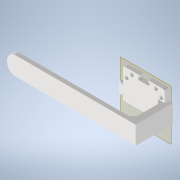
# Autodesk Inventor part: 40_Cube_XY_Table_Illumination_Arm
Saved by Autodesk Inventor 2022 (Build 260153000, 153)
## iProperties
Created: 2022-09-09
Part Number: 40_Cube_XY_Table_Illumination_Arm
Material: Generisch
Document SubType Name: Modeling
Designer: UC2
Density: 1 g/cm^3
Appearance: Vorgabe
Author: UC2
Autodesk Inventor part; units mm, degrees
ref_plane "YZ Plane" through (0, 0, 0) normal (1, 0, 0) x (0, 1, 0)
ref_plane "XZ Plane" through (0, 0, 0) normal (0, 1, 0) x (-1, 0, 0)
ref_plane "XY Plane" through (0, 0, 0) normal (0, 0, 1) x (1, 0, 0)
ref_plane "Arbeitsebene1" through (0, 0, 0) normal (0, 0, 1) x (1, 0, 0)
sketch "Skizze1" plane through (0, 0, 0) normal (0, 0, 1) x (1, 0, 0)
  circle A0 centre (-6.0705, 15.2895) radius 3.5 projected
  circle A1 centre (15.2895, -6.0705) radius 3.5 projected
  line L0 (30.5395, 32.5395) -> (0.0395, 32.5395) projected
  arc A2 (32.5395, 30.5395) -> (30.5395, 32.5395) centre (30.5395, 30.5395) ccw projected
  line L1 (32.5395, 30.5395) -> (32.5395, 0.0395) projected
  arc A3 (30.5395, -1.9605) -> (32.5395, 0.0395) centre (30.5395, 0.0395) ccw projected
  line L2 (0.0395, -1.9605) -> (30.5395, -1.9605) projected
  arc A4 (-1.9605, 0.0395) -> (0.0395, -1.9605) centre (0.0395, 0.0395) ccw projected
  line L3 (-1.9605, 0.0395) -> (-1.9605, 30.5395) projected
  arc A5 (0.0395, 32.5395) -> (-1.9605, 30.5395) centre (0.0395, 30.5395) ccw projected
  circle A6 centre (-4.7105, -4.7105) radius 2.45 projected
  circle A7 centre (0.7895, -5.5105) radius 2.3 projected
  circle A8 centre (-5.5105, 0.7895) radius 2.3 projected
  circle A9 centre (-5.5105, 29.7895) radius 2.3 projected
  circle A10 centre (0.7895, 36.0895) radius 2.3 projected
  circle A11 centre (-4.7105, 35.2895) radius 2.45 projected
  circle A12 centre (36.0895, 0.7895) radius 2.3 projected
  circle A13 centre (29.7895, -5.5105) radius 2.3 projected
  circle A14 centre (35.2895, -4.7105) radius 2.45 projected
  circle A15 centre (36.0895, 29.7895) radius 2.3 projected
  circle A16 centre (29.7895, 36.0895) radius 2.3 projected
  circle A17 centre (35.2895, 35.2895) radius 2.45 projected
  line L4 (20.4019, 40.2895) -> (20.4019, 39.1582) projected
  arc A18 (20.4019, 39.1582) -> (20.6778, 38.7524) centre (20.7437, 39.0939) ccw projected
  arc A19 (20.2895, 34.6895) -> (20.6778, 38.7524) centre (20.2895, 36.7395) ccw projected
  line L5 (20.2895, 34.6895) -> (10.1895, 34.6895) projected
  arc A20 (9.8548, 38.762) -> (10.1895, 34.6895) centre (10.1895, 36.7395) ccw projected
  arc A21 (9.8548, 38.762) -> (10.1895, 39.1567) centre (9.7895, 39.1567) ccw projected
  line L6 (10.1895, 39.1567) -> (10.1895, 40.2895) projected
  line L7 (10.1895, 40.2895) -> (-7.7105, 40.2895) projected
  arc A22 (-7.7105, 40.2895) -> (-9.7105, 38.2895) centre (-7.7105, 38.2895) ccw projected
  line L8 (-9.7105, 20.2895) -> (-9.7105, 38.2895) projected
  line L9 (-10.8433, 20.2895) -> (-9.7105, 20.2895) projected
  arc A23 (-11.3366, 20.7079) -> (-10.8433, 20.2895) centre (-10.8433, 20.7895) ccw projected
  arc A24 (-11.3366, 20.7079) -> (-15.2105, 20.3895) centre (-13.2605, 20.3895) ccw projected
  line L10 (-15.2105, 10.2895) -> (-15.2105, 20.3895) projected
  arc A25 (-15.2105, 10.2895) -> (-11.3515, 9.8916) centre (-13.2605, 10.2895) ccw projected
  arc A26 (-10.862, 10.2895) -> (-11.3515, 9.8916) centre (-10.862, 9.7895) ccw projected
  line L11 (-9.7105, 10.2895) -> (-10.862, 10.2895) projected
  line L12 (-9.7105, -7.7105) -> (-9.7105, 10.2895) projected
  arc A27 (-9.7105, -7.7105) -> (-7.7105, -9.7105) centre (-7.7105, -7.7105) ccw projected
  line L13 (-7.7105, -9.7105) -> (10.2895, -9.7105) projected
  line L14 (10.2895, -10.8433) -> (10.2895, -9.7105) projected
  arc A28 (9.8712, -11.3366) -> (10.2895, -10.8433) centre (9.7895, -10.8433) ccw projected
  arc A29 (9.8712, -11.3366) -> (10.1895, -15.2105) centre (10.1895, -13.2605) ccw projected
  line L15 (20.2895, -15.2105) -> (10.1895, -15.2105) projected
  arc A30 (20.2895, -15.2105) -> (20.6875, -11.3515) centre (20.2895, -13.2605) ccw projected
  arc A31 (20.2895, -10.862) -> (20.6875, -11.3515) centre (20.7895, -10.862) ccw projected
  line L16 (20.2895, -9.7105) -> (20.2895, -10.862) projected
  line L17 (20.2895, -9.7105) -> (38.2895, -9.7105) projected
  arc A32 (38.2895, -9.7105) -> (40.2895, -7.7105) centre (38.2895, -7.7105) ccw projected
  line L18 (40.2895, 10.1772) -> (40.2895, -7.7105) projected
  line L19 (40.2895, 10.1772) -> (39.1582, 10.1772) projected
  arc A33 (39.1582, 10.1772) -> (38.7524, 9.9013) centre (39.0939, 9.8354) ccw projected
  arc A34 (34.6895, 10.2895) -> (38.7524, 9.9013) centre (36.7395, 10.2895) ccw projected
  line L20 (34.6895, 10.2895) -> (34.6895, 20.3895) projected
  arc A35 (38.762, 20.7242) -> (34.6895, 20.3895) centre (36.7395, 20.3895) ccw projected
  arc A36 (38.762, 20.7242) -> (39.1567, 20.3895) centre (39.1567, 20.7895) ccw projected
  line L21 (39.1567, 20.3895) -> (40.2895, 20.3895) projected
  line L22 (40.2895, 38.2895) -> (40.2895, 20.3895) projected
  arc A37 (40.2895, 38.2895) -> (38.2895, 40.2895) centre (38.2895, 38.2895) ccw projected
  line L23 (38.2895, 40.2895) -> (20.4019, 40.2895) projected
  line L24 (40.2895, 26.3895) -> (45.2895, 26.3895)
  line L25 (45.2895, 26.3895) -> (45.2895, 4.1772)
  line L26 (45.2895, 4.1772) -> (40.2895, 4.1772)
  line L27 (40.2895, 4.1772) -> (40.2895, 26.3895)
  point P0 (0, 0)
  dimension "d0" = 5
  dimension "d2" = 6
  dimension "d3" = 6
  constraints: 8 end point, 2 parallel, 1 horizontal, 1 perpendicular, 1 point on line
  measures "d0" distance of L25.end L26.end
  measures "d2" distance of L21.end L24.start
  measures "d3" distance between parallel lines of L26 L19
extrude "Extrusion1" add sketch "Skizze1" along normal blind 5 contours A0 | A2 L1 A3 L2 A4 L3 A5 L0 | A6 | A11 | A14 | A17 | L23 A37 L22 L21 A36 A35 L20 A34 A33 L19 L18 A32 L17 L16 A31 A30 L15 A29 A28 L14 L13 A27 L12 L11 A26 A25 L10 A24 A23 L9 L8 A22 L7 L6 A21 A20 L5 A19 A18 L4 | L24 L25 L26 L18 L27 L22 | L27 L19 A33 A34 L20 A35 A36 L21
chamfer "Fase1" distance 1 angle 45 8 edges at (-1.5105, 36.0895, 0) (27.4895, 36.0895, 0) (33.7895, 29.7895, 0) (33.7895, 0.7895, 0) (27.4895, -5.5105, 0) (-1.5105, -5.5105, 0) (-7.8105, 0.7895, 0) (-7.8105, 29.7895, 0)
sketch "Skizze2" plane through (0, 0, 5) normal (0, 0, 1) x (1, 0, 0)
  line L0 (40.2895, 4.1772) -> (45.2895, 4.1772) projected
  line L1 (45.2895, 26.3895) -> (40.2895, 26.3895) projected
  line L2 (45.2895, 4.1772) -> (37.2895, 4.1772)
  line L3 (37.2895, 4.1772) -> (37.2895, 26.3895)
  line L4 (37.2895, 26.3895) -> (45.2895, 26.3895)
  line L5 (45.2895, 26.3895) -> (45.2895, 4.1772)
  point P0 (0, 0)
  point P1 (45.2895, 26.3895)
  point P2 (40.2895, 4.1772)
  dimension "d9" = 8
  constraints: 8 end point, 2 parallel, 1 horizontal, 1 perpendicular, 1 point on line
  measures "d9" distance of L3.end L4.end
extrude "Extrusion2" add sketch "Skizze2" along normal blind 45
sketch "Skizze3" plane through (0, 0, 50) normal (0, 0, 1) x (1, 0, 0)
  line L0 (45.2895, 26.3895) -> (37.2895, 26.3895) projected
  line L1 (37.2895, 26.3895) -> (37.2895, 4.1772) projected
  line L2 (37.2895, 4.1772) -> (45.2895, 4.1772) projected
  line L3 (45.2895, 4.1772) -> (45.2895, 26.3895) projected
  line L4 (45.2895, 26.3895) -> (37.2895, 26.3895) projected
  line L5 (37.2895, 26.3895) -> (-109.7105, 26.3895)
  line L6 (-109.7105, 26.3895) -> (-109.7105, 4.1772)
  line L7 (-109.7105, 4.1772) -> (37.2895, 4.1772)
  line L8 (37.2895, 4.1772) -> (37.2895, 26.3895)
  circle A0 centre (36.0895, 29.7895) radius 2.3 projected
  circle A1 centre (29.7895, -5.5105) radius 2.3 projected
  circle A2 centre (0.7895, 36.0895) radius 2.3 projected
  circle A3 centre (-5.5105, 29.7895) radius 2.3 projected
  circle A4 centre (-5.5105, 0.7895) radius 2.3 projected
  circle A5 centre (0.7895, -5.5105) radius 2.3 projected
  circle A6 centre (15.2895, -6.0705) radius 3.5 projected
  circle A7 centre (36.0895, 0.7895) radius 2.3 projected
  circle A8 centre (29.7895, 36.0895) radius 2.3 projected
  arc A9 (40.2895, 38.2895) -> (38.2895, 40.2895) centre (38.2895, 38.2895) ccw projected
  line L9 (38.2895, 40.2895) -> (20.4019, 40.2895) projected
  line L10 (20.4019, 40.2895) -> (20.4019, 39.1582) projected
  arc A10 (20.4019, 39.1582) -> (20.6778, 38.7524) centre (20.7437, 39.0939) ccw projected
  arc A11 (20.2895, 34.6895) -> (20.6778, 38.7524) centre (20.2895, 36.7395) ccw projected
  line L11 (20.2895, 34.6895) -> (10.1895, 34.6895) projected
  arc A12 (9.8548, 38.762) -> (10.1895, 34.6895) centre (10.1895, 36.7395) ccw projected
  arc A13 (9.8548, 38.762) -> (10.1895, 39.1567) centre (9.7895, 39.1567) ccw projected
  line L12 (10.1895, 39.1567) -> (10.1895, 40.2895) projected
  line L13 (10.1895, 40.2895) -> (-7.7105, 40.2895) projected
  arc A14 (-7.7105, 40.2895) -> (-9.7105, 38.2895) centre (-7.7105, 38.2895) ccw projected
  line L14 (-9.7105, 38.2895) -> (-9.7105, 20.2895) projected
  line L15 (-9.7105, 20.2895) -> (-10.8433, 20.2895) projected
  arc A15 (-11.3366, 20.7079) -> (-10.8433, 20.2895) centre (-10.8433, 20.7895) ccw projected
  arc A16 (-11.3366, 20.7079) -> (-15.2105, 20.3895) centre (-13.2605, 20.3895) ccw projected
  line L16 (-15.2105, 20.3895) -> (-15.2105, 10.2895) projected
  arc A17 (-15.2105, 10.2895) -> (-11.3515, 9.8916) centre (-13.2605, 10.2895) ccw projected
  arc A18 (-10.862, 10.2895) -> (-11.3515, 9.8916) centre (-10.862, 9.7895) ccw projected
  line L17 (-10.862, 10.2895) -> (-9.7105, 10.2895) projected
  line L18 (-9.7105, 10.2895) -> (-9.7105, -7.7105) projected
  arc A19 (-9.7105, -7.7105) -> (-7.7105, -9.7105) centre (-7.7105, -7.7105) ccw projected
  line L19 (-7.7105, -9.7105) -> (10.2895, -9.7105) projected
  line L20 (10.2895, -9.7105) -> (10.2895, -10.8433) projected
  arc A20 (9.8712, -11.3366) -> (10.2895, -10.8433) centre (9.7895, -10.8433) ccw projected
  arc A21 (9.8712, -11.3366) -> (10.1895, -15.2105) centre (10.1895, -13.2605) ccw projected
  line L21 (10.1895, -15.2105) -> (20.2895, -15.2105) projected
  arc A22 (20.2895, -15.2105) -> (20.6875, -11.3515) centre (20.2895, -13.2605) ccw projected
  arc A23 (20.2895, -10.862) -> (20.6875, -11.3515) centre (20.7895, -10.862) ccw projected
  line L22 (20.2895, -10.862) -> (20.2895, -9.7105) projected
  line L23 (20.2895, -9.7105) -> (38.2895, -9.7105) projected
  arc A24 (38.2895, -9.7105) -> (40.2895, -7.7105) centre (38.2895, -7.7105) ccw projected
  line L24 (40.2895, -7.7105) -> (40.2895, 4.1772) projected
  line L25 (37.2895, 4.1772) -> (37.2895, 26.3895) projected
  line L26 (40.2895, 26.3895) -> (40.2895, 38.2895) projected
  line L27 (37.2895, 26.3895) -> (40.2895, 26.3895) projected
  line L28 (40.2895, 4.1772) -> (37.2895, 4.1772) projected
  point P0 (0, 0)
  dimension "d24" = 100
  constraints: 8 end point, 2 parallel, 1 horizontal, 1 perpendicular
  measures "d24" distance between parallel lines of L14 L6
extrude "Extrusion3" add sketch "Skizze3" along normal blind 5 contours L3 L2 L1 L0 | L1 L7 L18 L17 A18 A17 L16 A16 A15 L15 L14 L5 | L14 L15 A15 A16 L16 A17 A18 L17 L18 L7 L6 L5
chamfer "Fase2" distance 10 angle 45 1 edges at (37.2895, 15.2834, 50)
sketch "Skizze5" plane through (0, 0, 5) normal (0, 0, 1) x (1, 0, 0)
  line L0 (-109.7105, 4.1772) -> (45.2895, 4.1772) projected
  line L1 (45.2895, 4.1772) -> (45.2895, 26.3895) projected
  line L2 (45.2895, 26.3895) -> (-109.7105, 26.3895) projected
  line L3 (-109.7105, 26.3895) -> (-109.7105, 4.1772) projected
  line L4 (-109.7105, 4.1772) -> (45.2895, 4.1772) projected
  line L5 (-38.4596, 4.1772) -> (42.3638, 4.1772)
  line L6 (42.3638, 4.1772) -> (42.3638, -19.3333)
  line L7 (42.3638, -19.3333) -> (-38.4596, -19.3333)
  line L8 (-38.4596, -19.3333) -> (-38.4596, 4.1772)
  point P0 (0, 0)
  point P1 (-38.4596, 4.1772)
  point P2 (-38.4596, 4.1772)
  constraints: 8 end point, 2 parallel, 1 horizontal, 1 perpendicular, 1 point on line
extrude "Extrusion5" cut sketch "Skizze5" against normal blind 10 contours L0 L6 L7 L8
fillet "Rundung1" radius 10 2 edges at (-109.7105, 4.1772, 52.5) (-109.7105, 26.3895, 52.5)
sketch "Skizze6" plane through (0, 0, 5) normal (0, 0, 1) x (1, 0, 0)
  circle A0 centre (36.0895, 29.7895) radius 2.3 projected
  circle A1 centre (0.7895, 36.0895) radius 2.3 projected
  circle A2 centre (-5.5105, 29.7895) radius 2.3 projected
  circle A3 centre (29.7895, 36.0895) radius 2.3 projected
  line L0 (-9.7105, 4.1772) -> (37.2895, 4.1772) projected
  line L1 (37.2895, 26.3895) -> (40.2895, 26.3895) projected
  line L2 (40.2895, 26.3895) -> (40.2895, 38.2895) projected
  arc A4 (40.2895, 38.2895) -> (38.2895, 40.2895) centre (38.2895, 38.2895) ccw projected
  line L3 (38.2895, 40.2895) -> (20.4019, 40.2895) projected
  line L4 (20.4019, 40.2895) -> (20.4019, 39.1582) projected
  arc A5 (20.4019, 39.1582) -> (20.6778, 38.7524) centre (20.7437, 39.0939) ccw projected
  arc A6 (20.2895, 34.6895) -> (20.6778, 38.7524) centre (20.2895, 36.7395) ccw projected
  line L5 (20.2895, 34.6895) -> (10.1895, 34.6895) projected
  arc A7 (9.8548, 38.762) -> (10.1895, 34.6895) centre (10.1895, 36.7395) ccw projected
  arc A8 (9.8548, 38.762) -> (10.1895, 39.1567) centre (9.7895, 39.1567) ccw projected
  line L6 (10.1895, 39.1567) -> (10.1895, 40.2895) projected
  line L7 (10.1895, 40.2895) -> (-7.7105, 40.2895) projected
  arc A9 (-7.7105, 40.2895) -> (-9.7105, 38.2895) centre (-7.7105, 38.2895) ccw projected
  line L8 (-9.7105, 38.2895) -> (-9.7105, 20.2895) projected
  line L9 (-9.7105, 20.2895) -> (-10.8433, 20.2895) projected
  arc A10 (-11.3366, 20.7079) -> (-10.8433, 20.2895) centre (-10.8433, 20.7895) ccw projected
  arc A11 (-11.3366, 20.7079) -> (-15.2105, 20.3895) centre (-13.2605, 20.3895) ccw projected
  line L10 (-15.2105, 20.3895) -> (-15.2105, 10.2895) projected
  arc A12 (-15.2105, 10.2895) -> (-11.3515, 9.8916) centre (-13.2605, 10.2895) ccw projected
  arc A13 (-10.862, 10.2895) -> (-11.3515, 9.8916) centre (-10.862, 9.7895) ccw projected
  line L11 (-10.862, 10.2895) -> (-9.7105, 10.2895) projected
  line L12 (-9.7105, 10.2895) -> (-9.7105, 4.1772) projected
  circle A14 centre (-20.2105, 36.0895) radius 2.6
  line L13 (20.4019, 40.2895) -> (10.1895, 40.2895)
  line L14 (-9.7105, 40.2895) -> (-17.6105, 40.2895)
  line L15 (-17.6105, 30.3395) -> (-17.6105, 4.1772)
  line L16 (-17.6105, 4.1772) -> (-9.7105, 4.1772)
  line L17 (-9.7105, 4.1772) -> (-9.7105, 40.2895)
  line L18 (-17.6105, 40.2895) -> (-22.6105, 40.2895)
  line L19 (-24.6105, 38.2895) -> (-24.6105, 34.3395)
  line L20 (-22.6105, 32.3395) -> (-19.6105, 32.3395)
  line L21 (-17.6105, 32.3395) -> (-17.6105, 40.2895)
  circle A15 centre (-14.7105, 35.2895) radius 2.425 projected
  circle A16 centre (-13.9105, 29.7895) radius 2.6 projected
  line L22 (27.2895, 4.1772) -> (37.2895, 4.1772) projected
  line L23 (37.2895, 4.1772) -> (37.2895, 26.3895) projected
  line L24 (37.2895, 26.3895) -> (27.2895, 26.3895) projected
  line L25 (27.2895, 26.3895) -> (27.2895, 4.1772) projected
  circle A17 centre (-13.7105, 15.6895) radius 2.5
  line L26 (37.2895, 4.1772) -> (37.2895, 26.3895) projected
  line L27 (-9.7105, 40.2895) -> (-7.7105, 40.2895)
  arc A18 (-22.6105, 40.2895) -> (-24.6105, 38.2895) centre (-22.6105, 38.2895) ccw
  arc A19 (-24.6105, 34.3395) -> (-22.6105, 32.3395) centre (-22.6105, 34.3395) ccw
  arc A20 (-17.6105, 30.3395) -> (-19.6105, 32.3395) centre (-19.6105, 30.3395) ccw
  point P0 (0, 0)
  point P1 (-24.6105, 32.3395)
  point P2 (-24.6105, 40.2895)
  point P3 (-17.6105, 32.3395)
  dimension "d25" = 7
  dimension "d28" = 2
  constraints: 20 end point, 7 point on circle, 6 point on line, 6 tangent, 5 centre point, 4 horizontal, 4 parallel, 2 equal radius, 2 perpendicular, 4 other
  measures "d25" distance of L21.start point (-24.61, 32.34)
  measures "d28" radius of A18
extrude "Extrusion6" add sketch "Skizze6" along normal blind 5 contours L12 L17 L8 A9 L7 L6 A8 A7 L5 A6 A5 L4 L3 A4 L2 L1 L24 L25 L0 | L16 L15 A20 L20 A19 L19 A18 L18 L14 L17 L8 L9 A10 A11 L10 A17 A12 A13 L11 L12 | L25 L24 L23 L0 | L11 A13 A12 L10 A17 A11 A10 L9 L17 | L17 L27 A9 | L13 L4 A5 A6 L5 A7 A8 L6 | A15 | A16
